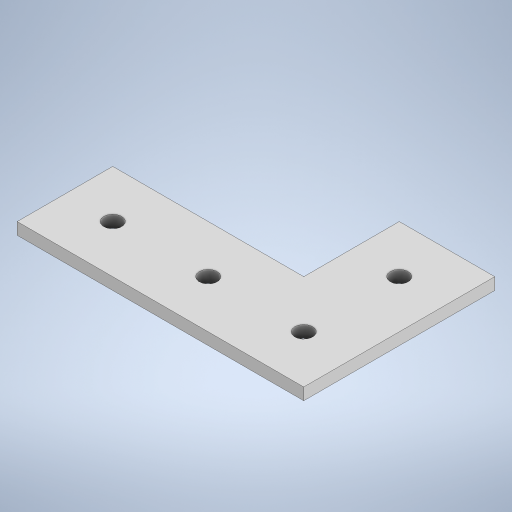
# Autodesk Inventor part: LPlate
Saved by Autodesk Inventor 2023.1 (Build 271208000, 208)
## iProperties
Created: 2022-07-20
Part Number: LPlate
Material: Generic
Document SubType Name: Modeling
Designer: Robotics
Density: 1 g/cm^3
Appearance: Default
Author: Robotics
Autodesk Inventor part; units mm, degrees
ref_plane "YZ Plane" through (0, 0, 0) normal (1, 0, 0) x (0, 1, 0)
ref_plane "XZ Plane" through (0, 0, 0) normal (0, 1, 0) x (-1, 0, 0)
ref_plane "XY Plane" through (0, 0, 0) normal (0, 0, 1) x (1, 0, 0)
sketch "Sketch1" plane through (0, 0, 0) normal (0, 1, 0) x (-1, 0, 0)
  line L0 (0, 0) -> (76.2, 0)
  line L1 (76.2, 0) -> (76.2, -25.4)
  line L2 (76.2, -25.4) -> (25.4, -25.4)
  line L3 (25.4, -25.4) -> (25.4, -50.8)
  line L4 (25.4, -50.8) -> (0, -50.8)
  line L5 (0, -50.8) -> (0, 0)
  line L6 (0, 0) -> (0, -12.7)
  line L7 (0, -12.7) -> (12.7, -12.7)
  circle A0 centre (12.7, -12.7) radius 2.3813
  line L8 (12.7, -12.7) -> (12.7, -38.1)
  circle A1 centre (12.7, -38.1) radius 2.3812
  line L9 (12.7, -12.7) -> (38.1, -12.7)
  circle A2 centre (38.1, -12.7) radius 2.3812
  line L10 (38.1, -12.7) -> (63.5, -12.7)
  circle A3 centre (63.5, -12.7) radius 2.3813
  dimension "d9" = 76.2
  dimension "d10" = 25.4
  dimension "d11" = 50.8
  dimension "d12" = 25.4
  dimension "d13" = 25.4
  dimension "d14" = 50.8
  dimension "d15" = 12.7
  dimension "d16" = 12.7
  dimension "d17" = 4.7625
  dimension "d18" = 25.4
  dimension "d19" = 4.7625
  dimension "d20" = 25.4
  dimension "d21" = 4.7625
  dimension "d22" = 25.4
  dimension "d23" = 4.7625
  constraints: 22 end point, 5 perpendicular, 4 centre point, 4 coincident, 3 horizontal, 1 point on line, 1 vertical
  measures "d9" distance of L0.start L0.end
  measures "d10" distance of L0.end L1.end
  measures "d11" distance of L1.end L2.end
  measures "d12" distance of L2.end L3.end
  measures "d13" distance of L3.end L4.end
  measures "d14" distance of L4.end L0.start
  measures "d15" distance of L0.start L6.end
  measures "d16" distance of L6.end L7.end
  measures "d17" diameter of A0
  measures "d18" distance of L8.start L8.end
  measures "d19" diameter of A1
  measures "d20" distance of L8.start L9.end
  measures "d21" diameter of A2
  measures "d22" distance of L10.start L10.end
  measures "d23" diameter of A3
extrude "Extrusion1" add sketch "Sketch1" along normal blind 3.175
body "Solid1"
